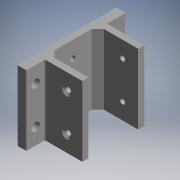
# Autodesk Inventor part: 6825_p
Saved by Autodesk Inventor 2017.3 (Build 213256000, 256)
## iProperties
Part Number: 6825_p
Material: Generic
Catalog Web Link: www.cadenas.de
Description: 6725, 6425, 6726, 6426, 6825, 6525, 6826, 6526_p-Double Flange Linear Bearings
Vendor: 8020
Document SubType Name: Modeling
Designer: partserver
Manufacturer: 8020
Mass: 91.8674 g
Surface Area: 300.205 cm^2
Volume: 91.8674 cm^3
Density: 1 g/cm^3
Appearance: PSOLRGB-191-191-191
Category: PARTsolutions
Company: 8020
Title: 6825_p
Author: Cadenas PARTsolutions
Comments: Double Flange Linear Bearings
PSOL_IDENT_0: {$CADENAS_DATA\23d-libs\8020\inch\linear_motion\6725.prj},194 {VTYP=3D},{NB=6825_p},{LINA=6825_p},{N
PSOL_IDENT_1: N=6725, 6425, 6726, 6426, 6825, 6525, 6826, 6526_p},{DATE=31.07.2020 09:21:20},{GEOMDATE=19.09.2017
PSOL_IDENT_2: 12:19:39},{VERSION=},{LINEID=50},{WBVAR=},{WBNUMERIC=}  {NB=6825_p},{LINA=6825_p},{KT=DUMMY},{PN=682
PSOL_IDENT_3: 5},{A=1.500},{B=0.500},{C=2.500},{D=0.625},{E=1.250},{F=0.375},{G=4.000},{H=0.750},{J=3.250},{K=1.25
PSOL_IDENT_4: 0},{L=1.875},{M=1.500},{N=2.812},{P=0.656},{Q=0.000},{R=0.375},{S=0.125},{W=.665},{TH=0.250},{HD=0.3
PSOL_IDENT_5: 28},{CS=0.385},{HD1=0.201},{Z=0},{SCR=10-24},{NO=1},{COLOR=.75,.75,.75}
NB: 6825_p
NN: 6725, 6425, 6726, 6426, 6825, 6525, 6826, 6526_p
NT: Double Flange Linear Bearings
NBSYN: $PN._p
LINA: 6825_p
CATALOG: 80/20
PN: 6825
A: 1.5
B: 0.5
C: 2.5
D: 0.625
E: 1.25
F: 0.375
G: 4
H: 0.75
J: 3.25
K: 1.25
L: 1.875
M: 1.5
N: 2.812
P: 0.656
Q: 0
R: 0.375
S: 0.125
W: .665
SCR: 10-24
COLOR: .75,.75,.75
SUPPLIER: 8020
ARTICLENO: 6825_p
BOMINFO: 6825_p
CREATOR: CADENAS GmbH
Autodesk Inventor part; units mm, degrees
sketch "Sketch_1" plane through (0, 0, 0) normal (0, 0, 1) x (1, 0, 0)
  line L0 (-15.875, -25.4) -> (-15.875, -31.75)
  line L1 (-15.875, -31.75) -> (21.59, -31.75)
  line L2 (21.59, -31.75) -> (22.225, -32.385)
  line L3 (22.225, -32.385) -> (22.225, -50.165)
  line L4 (22.225, -50.165) -> (22.86, -50.8)
  line L5 (22.86, -50.8) -> (31.115, -50.8)
  line L6 (31.115, -50.8) -> (31.75, -50.165)
  line L7 (31.75, -50.165) -> (31.75, 50.165)
  line L8 (31.75, 50.165) -> (31.115, 50.8)
  line L9 (31.115, 50.8) -> (22.86, 50.8)
  line L10 (22.86, 50.8) -> (22.225, 50.165)
  line L11 (22.225, 50.165) -> (22.225, 32.385)
  line L12 (22.225, 32.385) -> (21.59, 31.75)
  line L13 (21.59, 31.75) -> (-15.875, 31.75)
  line L14 (-15.875, 31.75) -> (-15.875, 25.4)
  line L15 (-15.875, 25.4) -> (19.05, 25.4)
  line L16 (19.05, 25.4) -> (25.4, 19.05)
  line L17 (25.4, 19.05) -> (25.4, -19.05)
  line L18 (25.4, -19.05) -> (19.05, -25.4)
  line L19 (19.05, -25.4) -> (-15.875, -25.4)
  constraints: 40 end point
extrude "Extrusion1" add sketch "Sketch_1" along normal mid plane 71.4248
sketch "Sketch2" plane through (31.75, -50.165, 35.7124) normal (1, 0, 0) x (0, 0, -1)
  point P0 (16.6624, 91.44)
hole "Hole1" at (31.75, 41.275, 19.05) direction (-1, 0, 0) diameter 8.3312 depth 9.525
pattern_linear "Rectangular Pattern1" count 2 spacing 38.1 along (0, 0, -1) count 2 spacing 82.55 along (0, -1, 0) of "Hole1"
sketch "Sketch3" plane through (31.75, -50.165, 35.7124) normal (1, 0, 0) x (0, 0, -1)
  point P0 (16.6624, 50.165)
hole "Hole2" at (31.75, 0, 19.05) direction (-1, 0, 0) diameter 5.1054 depth 6.35 countersink diameter 9.779 countersink angle 100
pattern_linear "Rectangular Pattern2" count 2 spacing 38.1 along (0, 0, -1) of "Hole2"
sketch "Sketch4" plane through (-15.875, 31.75, 35.7124) normal (0, 1, 0) x (1, 0, 0)
  point P0 (15.875, 16.6624)
hole "Hole3" at (0, 31.75, 19.05) direction (0, -1, 0) diameter 5.1054 depth 6.35 countersink diameter 9.779 countersink angle 100
pattern_linear "Rectangular Pattern3" count 2 spacing 38.1 along (0, 0, -1) of "Hole3"
sketch "Sketch5" plane through (-15.875, -31.75, 35.7124) normal (0, -1, 0) x (1, 0, 0)
  point P0 (15.875, -16.6624)
hole "Hole4" at (0, -31.75, 19.05) direction (0, 1, 0) diameter 5.1054 depth 6.35 countersink diameter 9.779 countersink angle 100
pattern_linear "Rectangular Pattern4" count 2 spacing 38.1 along (0, 0, -1) of "Hole4"
ref_plane "s1_XY" through (25.4, 0, 19.05) normal (1, 0, 0) x (0, 0, -1)
ref_plane "s1_YZ" through (25.4, 0, 19.05) normal (0, 0, -1) x (0, 1, 0)
ref_plane "s1_ZX" through (25.4, 0, 19.05) normal (0, 1, 0) x (1, 0, 0)
ref_plane "s1_2_XY" through (25.4, 0, -19.05) normal (1, 0, 0) x (0, 0, -1)
ref_plane "s1_2_YZ" through (25.4, 0, -19.05) normal (0, 0, -1) x (0, 1, 0)
ref_plane "s1_2_ZX" through (25.4, 0, -19.05) normal (0, 1, 0) x (1, 0, 0)
ref_plane "s2_XY" through (0, 25.4, 19.05) normal (0, 1, 0) x (1, 0, 0)
ref_plane "s2_YZ" through (0, 25.4, 19.05) normal (1, 0, 0) x (0, 0, -1)
ref_plane "s2_ZX" through (0, 25.4, 19.05) normal (0, 0, -1) x (0, 1, 0)
ref_plane "s2_2_XY" through (0, 25.4, -19.05) normal (0, 1, 0) x (1, 0, 0)
ref_plane "s2_2_YZ" through (0, 25.4, -19.05) normal (1, 0, 0) x (0, 0, -1)
ref_plane "s2_2_ZX" through (0, 25.4, -19.05) normal (0, 0, -1) x (0, 1, 0)
ref_plane "s3_XY" through (0, -25.4, 19.05) normal (0, 1, 0) x (1, 0, 0)
ref_plane "s3_YZ" through (0, -25.4, 19.05) normal (1, 0, 0) x (0, 0, -1)
ref_plane "s3_ZX" through (0, -25.4, 19.05) normal (0, 0, -1) x (0, 1, 0)
ref_plane "s3_2_XY" through (0, -25.4, -19.05) normal (0, 1, 0) x (1, 0, 0)
ref_plane "s3_2_YZ" through (0, -25.4, -19.05) normal (1, 0, 0) x (0, 0, -1)
ref_plane "s3_2_ZX" through (0, -25.4, -19.05) normal (0, 0, -1) x (0, 1, 0)
ref_plane "t1_1_XY" through (29.7892, 0, 19.05) normal (1, 0, 0) x (0, 0, -1)
ref_plane "t1_1_YZ" through (29.7892, 0, 19.05) normal (0, 0, -1) x (0, 1, 0)
ref_plane "t1_1_ZX" through (29.7892, 0, 19.05) normal (0, 1, 0) x (1, 0, 0)
ref_plane "t1_2_XY" through (29.7892, 0, -19.05) normal (1, 0, 0) x (0, 0, -1)
ref_plane "t1_2_YZ" through (29.7892, 0, -19.05) normal (0, 0, -1) x (0, 1, 0)
ref_plane "t1_2_ZX" through (29.7892, 0, -19.05) normal (0, 1, 0) x (1, 0, 0)
ref_plane "t2_1_XY" through (0, 29.7892, 19.05) normal (0, 1, 0) x (1, 0, 0)
ref_plane "t2_1_YZ" through (0, 29.7892, 19.05) normal (1, 0, 0) x (0, 0, -1)
ref_plane "t2_1_ZX" through (0, 29.7892, 19.05) normal (0, 0, -1) x (0, 1, 0)
ref_plane "t2_2_XY" through (0, 29.7892, -19.05) normal (0, 1, 0) x (1, 0, 0)
ref_plane "t2_2_YZ" through (0, 29.7892, -19.05) normal (1, 0, 0) x (0, 0, -1)
ref_plane "t2_2_ZX" through (0, 29.7892, -19.05) normal (0, 0, -1) x (0, 1, 0)
ref_plane "t3_1_XY" through (0, -29.7892, 19.05) normal (0, 1, 0) x (1, 0, 0)
ref_plane "t3_1_YZ" through (0, -29.7892, 19.05) normal (1, 0, 0) x (0, 0, -1)
ref_plane "t3_1_ZX" through (0, -29.7892, 19.05) normal (0, 0, -1) x (0, 1, 0)
ref_plane "t3_2_XY" through (0, -29.7892, -19.05) normal (0, 1, 0) x (1, 0, 0)
ref_plane "t3_2_YZ" through (0, -29.7892, -19.05) normal (1, 0, 0) x (0, 0, -1)
ref_plane "t3_2_ZX" through (0, -29.7892, -19.05) normal (0, 0, -1) x (0, 1, 0)
body "Solid1"
